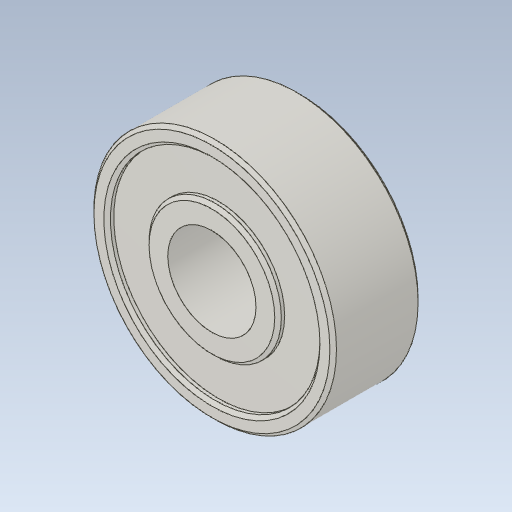
# Autodesk Inventor part: roller bearing
Saved by Autodesk Inventor 2020 (Build 240168000, 168)
## iProperties
Created: 2018-11-16
Part Number: roller bearing
Material: Steel AISI 1118
Document SubType Name: Modeling
Designer: LillaHunden
Density: 7.85 g/cm^3
Appearance: Steel
Mass: 2.37413 g
Surface Area: 3.67957 cm^2
Volume: 0.302436 cm^3
Author: LillaHunden
Autodesk Inventor part; units mm, degrees
ref_plane "YZ Plane" through (0, 0, 0) normal (1, 0, 0) x (0, 1, 0)
ref_plane "XZ Plane" through (0, 0, 0) normal (0, 1, 0) x (-1, 0, 0)
sketch "Sketch1" plane through (0, 0, 0) normal (0, 0, 1) x (1, 0, 0)
  circle A0 centre (0, 0) radius 5.5
  dimension "d0" = 11
  constraints: 1 centre point, 1 coincident
  measures "d0" diameter of A0
extrude "Extrusion1" add sketch "Sketch1" along normal blind 4
sketch "Sketch2" plane through (0, 0, 4) normal (0, 0, 1) x (1, 0, 0)
  circle A0 centre (0, 0) radius 2
  dimension "d3" = 4
  constraints: 1 centre point, 1 coincident
  measures "d3" diameter of A0
extrude "Extrusion2" cut sketch "Sketch2" against normal blind 4
sketch "Sketch3" plane through (0, 0, 4) normal (0, 0, 1) x (1, 0, 0)
  circle A0 centre (0, 0) radius 2 projected
  circle A1 centre (0, 0) radius 3
  circle A2 centre (0, 0) radius 4.75
  dimension "d6" = 1
  dimension "d7" = 9.5
  constraints: 2 centre point, 1 coincident
  measures "d6" radial gap between concentric circles of A0 A1
  measures "d7" diameter of A2
extrude "Extrusion3" cut sketch "Sketch3" against normal blind 0.3 contours A2
ref_plane "Work Plane1" through (0, 0, 2) normal (0, 0, 1) x (1, 0, 0)
mirror "Mirror1" about plane through (0, 0, 2) normal (0, 0, 1) of "Extrusion3"
chamfer "Chamfer1" distance 0.15 angle 45 6 edges at (-4.75, 0, 4) (-3, 0, 4) (-3, 0, 0) (-4.75, 0, 0) (-5.5, 0, 4) (-5.5, 0, 0)
body "Solid1"
